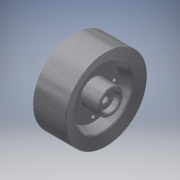
# Autodesk Inventor part: Wheel Hub
Saved by Autodesk Inventor 2018 (Build 220112000, 112)
## iProperties
Created: 2018-08-07
Part Number: Wheel Hub
Material: Generic
Document SubType Name: Modeling
Designer: ruben
Density: 1 g/cm^3
Appearance: Aluminum Cast
Author: ruben
Autodesk Inventor part; units mm, degrees
ref_plane "YZ Plane" through (0, 0, 0) normal (1, 0, 0) x (0, 1, 0)
ref_plane "XZ Plane" through (0, 0, 0) normal (0, 1, 0) x (-1, 0, 0)
ref_plane "XY Plane" through (0, 0, 0) normal (0, 0, 1) x (1, 0, 0)
sketch "Sketch1" plane through (0, 0, 0) normal (0, 1, 0) x (-1, 0, 0)
  line L0 (4.95, 0) -> (-68.2, 0) projected
  line L1 (0, -41.44) -> (0, 41.44) projected
  line L2 (-13, -29.6) -> (-17.75, -29.6)
  line L3 (-17.75, 29.6) -> (-13, 29.6)
  line L4 (-17.75, -4.6) -> (-36.75, -4.6)
  line L5 (-36.75, -4.6) -> (-41.75, -18.6)
  line L6 (-17.75, 4.6) -> (-36.75, 4.6)
  line L7 (-36.75, 4.6) -> (-41.75, 18.6)
  line L8 (-41.75, -18.6) -> (-57.75, -23.6)
  line L9 (-41.75, 18.6) -> (-57.75, 23.6)
  line L10 (-57.75, -23.6) -> (-57.75, 23.6)
  line L11 (-17.75, -29.6) -> (-17.75, -4.6)
  line L12 (-17.75, 4.6) -> (-17.75, 29.6)
  line L13 (-5.5, -21.5) -> (-5.5, 21.5)
  line L14 (-13, -21.5) -> (-5.5, -21.5)
  line L15 (-5.5, 21.5) -> (-13, 21.5)
  line L16 (-13, -29.6) -> (-13, -21.5)
  line L17 (-13, 21.5) -> (-13, 29.6)
  dimension "d0" = 59.2
  dimension "d4" = 19
  dimension "d5" = 19
  dimension "d6" = 25
  dimension "d8" = 14
  dimension "d9" = 5
  dimension "d10" = 14
  dimension "d11" = 5
  dimension "d12" = 16
  dimension "d13" = 16
  dimension "d14" = 5
  dimension "d15" = 5
  dimension "d16" = 35.5
  dimension "d18" = 11
  dimension "d19" = 43
  dimension "d20" = 4.75
  dimension "d21" = 4.75
  constraints: 32 end point, 7 parallel, 4 vertical, 2 horizontal, 2 perpendicular, 3 other
  measures "d0" distance of L2.start L3.end
  measures "d4" distance of L4.start L4.end
  measures "d5" distance of L6.start L6.end
  measures "d6" distance between parallel lines of L2 L4
  measures "d8" vertical distance of L5.end L4.end
  measures "d9" horizontal distance of L4.end L5.end
  measures "d10" vertical distance of L7.end L6.end
  measures "d11" horizontal distance of L6.end L7.end
  measures "d12" horizontal distance of L8.end L5.end
  measures "d13" horizontal distance of L9.end L7.end
  measures "d14" vertical distance of L7.end L9.end
  measures "d15" vertical distance of L5.end L8.end
  measures "d16" diameter of L11 L1
  measures "d18" diameter of L13 L1
  measures "d19" distance between parallel lines of L15 L14
  measures "d20" distance of L2.start L2.end
  measures "d21" distance of L3.start L3.end
revolve "Revolution1" add sketch "Sketch1" angle 360 about axis through (0, 0, -10) along (0, 0, 1)
chamfer "Chamfer1" distance 1 angle 45 9 edges at (-17.75, 0, 29.6) (-13, 0, 29.6) (-41.75, 0, 18.6) (-57.75, 0, 23.6) (-57.75, 0, -23.6) (-17.75, 0, -29.6) (-13, 0, -29.6) (-5.5, 0, -21.5) (-5.5, 0, 21.5)
sketch "Sketch3" plane through (0, 0, 4.6) normal (0, 0, 1) x (1, 0, 0)
  line L0 (-80.85, 0) -> (80.85, 0) projected
  line L1 (0, -80.85) -> (0, 80.85) projected
  point P0 (0, 0)
  point P1 (0, 30)
  dimension "d25" = 30
  constraints: 1 point on line
  measures "d25" distance of point (0, 30) point (0, 0)
hole "Hole1" at (0, 30, 4.6) direction (0, 0, -1) diameter 5 end through all
pattern_circular "Circular Pattern1" count 4 over 360 about axis through (0, 0, -10) along (0, 0, 1) of "Hole1"
equation "\"d5\" = d4"
equation "\"d10\" = d8"
equation "\"d11\" = d9"
equation "\"d13\" = d12"
equation "\"d14\" = d15"
equation "\"d21\" = d20"
body "Solid1"
